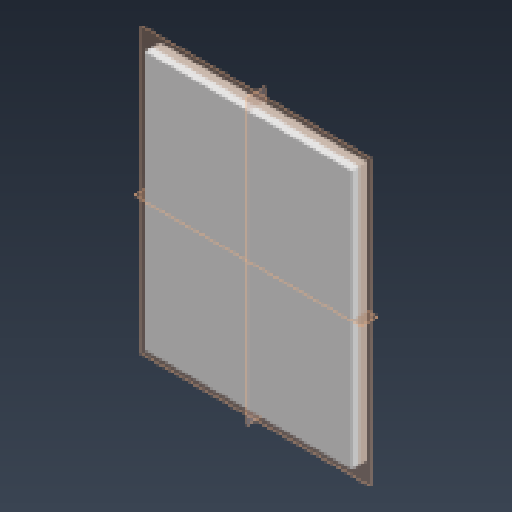
# Autodesk Inventor part: Фанерка_маркера
Saved by Autodesk Inventor 2023.2 (Build 272271030, 271C)
## iProperties
Created: 2026-01-04
Part Number: Фанерка_маркера
Material: Типовые
Document SubType Name: Modeling
Designer: Олег Коноваленко
Density: 1 g/cm^3
Appearance: По умолчанию
Author: Олег Коноваленко
Autodesk Inventor part; units mm, degrees
sketch "Эскиз1" plane through (0, 0, 0) normal (0, 0, 1) x (1, 0, 0)
  line L0 (-20, 25) -> (20, 25)
  line L1 (20, 25) -> (20, -25)
  line L2 (20, -25) -> (-20, -25)
  line L3 (-20, -25) -> (-20, 25)
  line L4 (-20, 25) -> (20, -25) construction
  line L5 (20, 25) -> (-20, -25) construction
  point P0 (0, 0)
  dimension "d0" = 50
  dimension "d1" = 40
  constraints: 12 end point, 2 midpoint, 2 parallel, 1 horizontal, 1 perpendicular
  measures "d0" distance of L0.end L1.end
  measures "d1" distance of L1.end L2.end
extrude "Выдавливание1" add sketch "Эскиз1" along normal mid plane 3
fillet "Сопряжение1" radius 5 4 edges at (20, -25, 0) (20, 25, 0) (-20, 25, 0) (-20, -25, 0)
